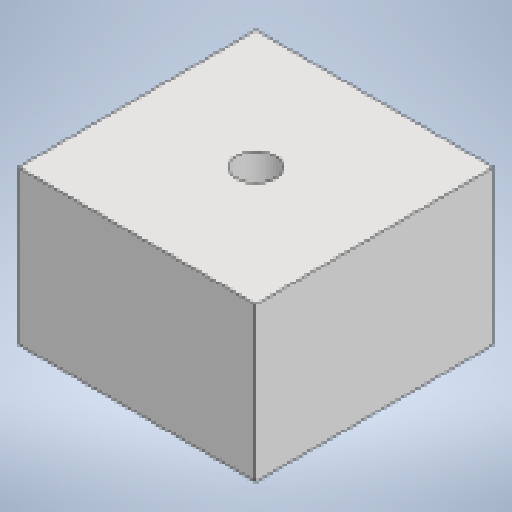
# Autodesk Inventor part: motor dummy
Saved by Autodesk Inventor 2025.1 (Build 291241020, 241B)
## iProperties
Created: 2024-12-05
Part Number: motor dummy
Material: Generic
Document SubType Name: Modeling
Designer: user
Density: 1 g/cm^3
Appearance: Default
Author: user
Autodesk Inventor part; units mm, degrees
ref_plane "YZ Plane" through (0, 0, 0) normal (1, 0, 0) x (0, 1, 0)
ref_plane "XZ Plane" through (0, 0, 0) normal (0, 1, 0) x (-1, 0, 0)
ref_plane "XY Plane" through (0, 0, 0) normal (0, 0, 1) x (1, 0, 0)
sketch "Sketch1" plane through (0, 0, 0) normal (0, 0, 1) x (1, 0, 0)
  line L0 (-85, 85) -> (85, 85)
  line L1 (85, 85) -> (85, -85)
  line L2 (85, -85) -> (-85, -85)
  line L3 (-85, -85) -> (-85, 85)
  line L4 (-85, 85) -> (85, -85) construction
  line L5 (85, 85) -> (-85, -85) construction
  circle A0 centre (0, 0) radius 14
  dimension "d0" = 170
  dimension "d1" = 170
  dimension "d2" = 28
  constraints: 12 end point, 2 midpoint, 2 parallel, 1 centre point, 1 coincident, 1 horizontal, 1 perpendicular
  measures "d0" distance of L1.end L2.end
  measures "d1" distance of L0.end L1.end
  measures "d2" diameter of A0
extrude "Extrusion1" add sketch "Sketch1" along normal blind 110
sketch "Sketch2" plane through (-85, 85, 0) normal (0, 1, 0) x (1, 0, 0)
  line L0 (170, 0) -> (0, 0) projected
  line L1 (0, 0) -> (0, -110) projected
  line L2 (170, -110) -> (0, -110) projected
  line L3 (170, 0) -> (170, -110) projected
  circle A0 centre (30.3826, -55) radius 73.696
  point P0 (85, 0)
  constraints: 1 centre point
extrude "Extrusion2" add sketch "Sketch2" along normal blind 271 contours A0 L2 L1 L0 | L0 L1 L2 A0
body "Solid1"
